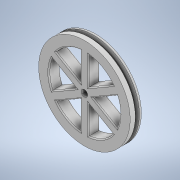
# Autodesk Inventor part: Wheel
Saved by Autodesk Inventor 2020 (Build 240168000, 168)
## iProperties
Created: 2019-08-13
Part Number: Wheel
Material: 일반
Document SubType Name: Modeling
Designer: Jeong Ji Hoon
Mass: 81.9381 g
Surface Area: 319.569 cm^2
Volume: 81.9381 cm^3
Density: 1 g/cm^3
Appearance: 기본값
Author: Jeong Ji Hoon
## iProperties of the stored document _3D 인쇄.ipt
Created: 2019-08-15
Part Number: _3D 인쇄
Material: 일반
Document SubType Name: Modeling
Designer: Jeong Ji Hoon
Density: 1 g/cm^3
Appearance: 기본값
Author: Jeong Ji Hoon
Autodesk Inventor part; units mm, degrees
ref_plane "YZ Plane" through (0, 0, 0) normal (1, 0, 0) x (0, 1, 0)
ref_plane "XZ Plane" through (0, 0, 0) normal (0, 1, 0) x (-1, 0, 0)
ref_plane "XY Plane" through (0, 0, 0) normal (0, 0, 1) x (1, 0, 0)
sketch "스케치1" plane through (0, 0, 0) normal (0, 0, 1) x (1, 0, 0)
  circle A0 centre (0, 0) radius 45
  dimension "d0" = 90
  constraints: 1 centre point, 1 coincident
  measures "d0" diameter of A0
extrude "돌출1" add sketch "스케치1" along normal blind 3
sketch "스케치2" plane through (0, 0, 3) normal (0, 0, 1) x (1, 0, 0)
  circle A0 centre (0, 0) radius 45 projected
  circle A1 centre (0, 0) radius 37.5
  dimension "d3" = 75
  constraints: 1 centre point, 1 coincident
  measures "d3" diameter of A1
extrude "돌출2" add sketch "스케치2" along normal blind 3 contours A1
sketch "스케치3" plane through (0, 0, 6) normal (0, 0, 1) x (1, 0, 0)
  circle A0 centre (0, 0) radius 37.5 projected
  circle A1 centre (0, 0) radius 45
  dimension "d6" = 90
  constraints: 1 centre point, 1 coincident
  measures "d6" diameter of A1
extrude "돌출3" add sketch "스케치3" along normal blind 5 contours A0 | A1
sketch "스케치4" plane through (0, 0, 11) normal (0, 0, 1) x (1, 0, 0)
  circle A0 centre (0, 0) radius 45 projected
  circle A1 centre (0, 0) radius 3.2
  line L0 (-2.5, -1.9975) -> (-2.5, 1.9975)
  circle A2 centre (0, 0) radius 35
  line L1 (4, 0) -> (-4, 0)
  line L2 (-4, 0) -> (-4, -35)
  line L3 (-4, -35) -> (4, -35)
  line L4 (4, -35) -> (4, 0)
  line L5 (32.3109, -14.0359) -> (2, 3.4641)
  line L6 (-2, -3.4641) -> (28.3109, -20.9641)
  line L7 (28.3109, -20.9641) -> (32.3109, -14.0359)
  line L8 (2, 3.4641) -> (-2, -3.4641)
  line L9 (28.3109, 20.9641) -> (-2, 3.4641)
  line L10 (2, -3.4641) -> (32.3109, 14.0359)
  line L11 (32.3109, 14.0359) -> (28.3109, 20.9641)
  line L12 (-2, 3.4641) -> (2, -3.4641)
  line L13 (-4, 35) -> (-4, 0)
  line L14 (4, 0) -> (4, 35)
  line L15 (4, 35) -> (-4, 35)
  line L16 (-4, 0) -> (4, 0)
  line L17 (-32.3109, 14.0359) -> (-2, -3.4641)
  line L18 (2, 3.4641) -> (-28.3109, 20.9641)
  line L19 (-28.3109, 20.9641) -> (-32.3109, 14.0359)
  line L20 (-2, -3.4641) -> (2, 3.4641)
  line L21 (-28.3109, -20.9641) -> (2, -3.4641)
  line L22 (-2, 3.4641) -> (-32.3109, -14.0359)
  line L23 (-32.3109, -14.0359) -> (-28.3109, -20.9641)
  line L24 (2, -3.4641) -> (-2, 3.4641)
  point P0 (32.1123, 13.9212)
  point P1 (8, 0)
  point P2 (32.1123, -13.9212)
  point P3 (4, 34.7707)
  point P4 (4, 6.9282)
  point P5 (28.1123, 20.8494)
  point P6 (-28.1123, 20.8494)
  point P7 (-4, 6.9282)
  point P8 (-4, 34.7707)
  point P9 (-32.1123, -13.9212)
  point P10 (-8, 0)
  point P11 (-32.1123, 13.9212)
  point P12 (-4, -6.9282)
  point P13 (-28.1123, -20.8494)
  point P14 (-4, -34.7707)
  point P15 (28.1123, -20.8494)
  point P16 (4, -6.9282)
  point P17 (4, -34.7707)
  point P18 (0, 0)
  point P19 (0, 0)
  point P20 (0, 0)
  point P21 (0, 0)
  point P22 (0, 0)
  point P23 (0, 0)
  dimension "d10" = 6.4
  dimension "d11" = 2.5
  dimension "d14" = 70
  dimension "d15" = 8
  dimension "d16" = 35
  dimension "d19" = 360
  constraints: 50 end point, 3 coincident, 2 centre point, 2 parallel, 2 point on circle, 1 horizontal, 1 midpoint, 1 perpendicular, 1 vertical, 55 other
  measures "d10" diameter of A1
  measures "d11" distance from line of L0 A0.centre
  measures "d14" diameter of A2
  measures "d15" distance of L1.start L1.end
  measures "d16" distance between parallel lines of L1 L3
extrude "돌출4" cut sketch "스케치4" against normal through all contours L1 L8 A1 | A1 L12 L1 | L8 L12 A1 | A1 L8 L12 | L8 A1 L0 L1 | L1 L0 A1 L12 | L6 A2 L4 | L10 A2 L5 | L14 A2 L9 | L18 A2 L13 | L2 A2 L21 | L22 A2 L17
fillet "모깎기2" radius 1 36 edges at (-20.0561, -6.9606, 11) (-16.0561, -13.8888, 11) (-35, 0, 11) (-20.0561, 6.9606, 11) (-16.0561, 13.8888, 11) (-17.5, 30.3109, 11) (-4, 20.8494, 11) (4, 20.8494, 11) (17.5, 30.3109, 11) (16.0561, 13.8888, 11) (20.0561, 6.9606, 11) (20.0561, 6.9606, 0) (35, 0, 11) (4, 20.8494, 0) (17.5, 30.3109, 0) (20.0561, -6.9606, 11) (16.0561, -13.8888, 11) (4, -20.8494, 11) (4, -20.8494, 0) (16.0561, -13.8888, 0) (-4, -20.8494, 11) (-16.0561, -13.8888, 0) (-20.0561, 6.9606, 0) (-17.5, 30.3109, 0) (-35, 0, 0) (-17.5, -30.3109, 0) (-17.5, -30.3109, 11) (-4, -20.8494, 0) (17.5, -30.3109, 11) (17.5, -30.3109, 0) (35, 0, 0) (20.0561, -6.9606, 0) (-4, 20.8494, 0) (-16.0561, 13.8888, 0) (16.0561, 13.8888, 0) (-20.0561, -6.9606, 0)
chamfer "모따기1" distance 3 distance2 1 1 edges at (-45, 0, 3) measured on face at (42.1722, 3.1187, 3)
